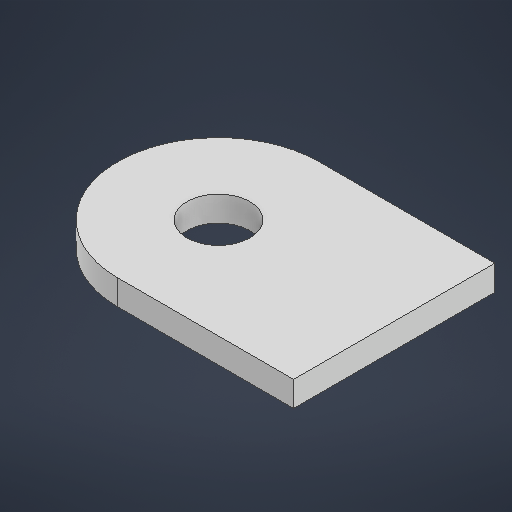
# Autodesk Inventor part: cup holder
Saved by Autodesk Inventor 2027 (Build 310192000, 192)
## iProperties
Created: 2026-04-25
Part Number: cup holder
Material: Generic
Document SubType Name: Modeling
Designer: ratik
Density: 1 g/cm^3
Appearance: Default
Author: ratik
Autodesk Inventor part; units mm, degrees
ref_plane "YZ Plane" through (0, 0, 0) normal (1, 0, 0) x (0, 1, 0)
ref_plane "XZ Plane" through (0, 0, 0) normal (0, 1, 0) x (-1, 0, 0)
ref_plane "XY Plane" through (0, 0, 0) normal (0, 0, 1) x (1, 0, 0)
sketch "Sketch1" plane through (0, 0, 0) normal (0, 1, 0) x (-1, 0, 0)
  line L0 (19.3579, 14.5943) -> (-8.5995, 14.5943)
  line L1 (-8.5995, 14.5943) -> (-8.5995, -17.4057)
  line L2 (-8.5995, -17.4057) -> (19.3579, -17.4057)
  arc A0 (19.3579, -17.4057) -> (19.3579, 14.5943) centre (19.3579, -1.4057) ccw
  point P0 (0, 0)
  dimension "d0" = 32
  dimension "d2" = 32
  dimension "d3" = 16
  constraints: 6 end point, 2 point on circle, 1 centre point, 1 horizontal, 1 parallel, 1 perpendicular
  measures "d0" distance of L0.end L1.end
  measures "d2" diameter of A0
  measures "d3" distance from line of L2 A0.centre
extrude "Extrusion1" add sketch "Sketch1" along normal blind 4
sketch "Sketch2" plane through (0, 4, 0) normal (0, 1, 0) x (1, 0, 0)
  arc A0 (-19.3579, 17.4057) -> (-19.3579, -14.5943) centre (-19.3579, 1.4057) ccw projected
  circle A1 centre (-19.3579, 1.4057) radius 5
  point P0 (0, 0)
  dimension "d6" = 10
  constraints: 1 centre point, 1 coincident
  measures "d6" diameter of A1
extrude "Extrusion2" cut sketch "Sketch2" against normal blind 4
body "Solid1"
